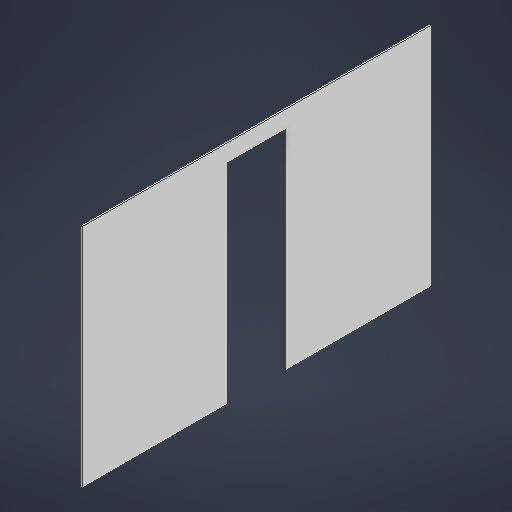
# Autodesk Inventor part: panel frontal
Saved by Autodesk Inventor 2027 (Build 310192060, 192F)
## iProperties
Created: 2026-09-04
Part Number: panel frontal
Material: Genérico
Document SubType Name: Modeling
Designer: Leandro
Density: 1 g/cm^3
Appearance: Valor por defecto
Author: Leandro
Autodesk Inventor part; units mm, degrees
ref_plane "YZ Plane" through (0, 0, 0) normal (1, 0, 0) x (0, 1, 0)
ref_plane "XZ Plane" through (0, 0, 0) normal (0, 1, 0) x (-1, 0, 0)
ref_plane "XY Plane" through (0, 0, 0) normal (0, 0, 1) x (1, 0, 0)
sketch "Boceto1" plane through (0, 0, 0) normal (1, 0, 0) x (0, 1, 0)
  line L0 (13.0609, 21.0882) -> (-181.9391, 21.0882)
  line L1 (-181.9391, -279.9118) -> (13.0609, -279.9118)
  line L2 (13.0609, -279.9118) -> (13.0609, 21.0882)
  line L3 (-1.9391, -129.4118) -> (-1.9391, -154.4118)
  line L4 (-1.9391, -154.4118) -> (-181.9391, -154.4118)
  line L5 (-1.9391, -129.4118) -> (-1.9391, -104.4118)
  line L6 (-1.9391, -104.4118) -> (-181.9391, -104.4118)
  line L7 (-181.9391, 21.0882) -> (-181.9391, -104.4118)
  line L8 (-181.9391, -154.4118) -> (-181.9391, -279.9118)
  point P0 (0, 0)
  dimension "d0" = 195
  dimension "d1" = 301
  dimension "d3" = 25
  dimension "d4" = 25
  constraints: 18 end point, 6 perpendicular, 3 parallel, 1 horizontal, 1 point on line
  measures "d0" distance of L1.end L1.start
  measures "d1" distance of L1.start L0.end
  measures "d3" distance of L3.start L3.end
  measures "d4" distance of L3.start L5.end
extrude "Extrusión1" add sketch "Boceto1" along normal mid plane 1.5
